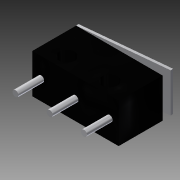
# Autodesk Inventor part: switch
Saved by Autodesk Inventor 2013 (Build 170138000, 138)
## iProperties
Created: 2013-09-11
Part Number: switch
Material: Generic
Document SubType Name: Modeling
Designer: employee
Density: 1 g/cm^3
Author: employee
Autodesk Inventor part; units mm, degrees
ref_plane "YZ Plane" through (0, 0, 0) normal (1, 0, 0) x (0, 1, 0)
ref_plane "XZ Plane" through (0, 0, 0) normal (0, 1, 0) x (-1, 0, 0)
ref_plane "XY Plane" through (0, 0, 0) normal (0, 0, 1) x (1, 0, 0)
sketch "Sketch1" plane through (0, 0, 0) normal (0, 0, 1) x (1, 0, 0)
  line L0 (0, 0) -> (12.827, 0)
  line L1 (12.827, 0) -> (12.827, 6.5278)
  line L2 (12.827, 6.5278) -> (0, 6.5278)
  line L3 (0, 6.5278) -> (0, 0)
  dimension "d0" = 12.827
  dimension "d2" = 6.5278
  constraints: 8 end point, 2 parallel, 1 coincident, 1 horizontal, 1 perpendicular
  measures "d0" distance of L0.start L0.end
  measures "d2" distance of L2.end L0.start
extrude "Extrusion1" add sketch "Sketch1" along normal blind 5.8
sketch "Sketch2" plane through (0, 0, 5.8) normal (0, 0, 1) x (1, 0, 0)
  line L0 (12.827, 6.5278) -> (0, 6.5278) projected
  line L1 (0, 6.5278) -> (12.764, 7.7978)
  line L2 (12.764, 7.7978) -> (12.7263, 8.1769)
  line L3 (12.7263, 8.1769) -> (-0.0377, 6.9069)
  line L4 (-0.0377, 6.9069) -> (0, 6.5278)
  dimension "d5" = 0.381
  dimension "d7" = 1.27
  constraints: 8 end point, 2 parallel, 1 equal length, 1 perpendicular
  measures "d5" distance between parallel lines of L3 L1
  measures "d7" vertical distance of L1.end L0.start
extrude "Extrusion2" add sketch "Sketch2" against normal up to surface (5.8 mm away)
sketch "Sketch3" plane through (0, 0, 0) normal (0, -1, 0) x (1, 0, 0)
  line L0 (12.827, 0) -> (12.827, 5.8) projected
  line L1 (0, 5.8) -> (12.827, 5.8) projected
  line L2 (0, 0) -> (0, 5.8) projected
  line L3 (1.3335, 2.9) -> (11.4935, 2.9)
  circle A0 centre (1.3335, 2.9) radius 0.4445
  circle A1 centre (6.4135, 2.9) radius 0.4445
  circle A2 centre (11.4935, 2.9) radius 0.4445
  point P0 (6.4135, 5.8)
  point P1 (12.827, 2.9)
  dimension "d10" = 10.16
  dimension "d12" = 0.889
  constraints: 3 centre point, 3 coincident, 3 midpoint, 2 end point, 2 equal radius, 1 horizontal alignment, 1 perpendicular, 1 vertical alignment
  measures "d10" distance of L3.start L3.end
  measures "d12" diameter of A2
extrude "Extrusion3" add sketch "Sketch3" along normal blind 3.81
sketch "Sketch4" plane through (0, 0, 5.8) normal (0, 0, 1) x (1, 0, 0)
  line L0 (0, 0) -> (12.827, 0) projected
  line L1 (0, 6.5278) -> (0, 0) projected
  line L2 (3.2385, 1.905) -> (9.5885, 1.905)
  circle A0 centre (3.2385, 1.905) radius 1.143
  circle A1 centre (9.5885, 1.905) radius 1.143
  point P0 (6.4135, 1.905)
  point P1 (6.4135, 0)
  dimension "d15" = 6.35
  dimension "d17" = 1.905
  dimension "d18" = 2.286
  constraints: 2 centre point, 2 coincident, 2 end point, 2 midpoint, 1 equal radius, 1 perpendicular, 1 vertical alignment
  measures "d15" distance of L2.start L2.end
  measures "d17" distance between parallel lines of L2 L0
  measures "d18" diameter of A1
extrude "Extrusion4" cut sketch "Sketch4" against normal through all
body "Solid1"
